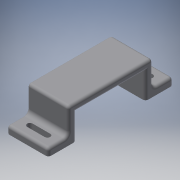
# Autodesk Inventor part: sujeta-taladro-0,1
Saved by Autodesk Inventor 2016 (Build 200138000, 138)
## iProperties
Created: 2015-03-20
Part Number: sujeta-taladro-0,1
Material: Generic
Document SubType Name: Modeling
Designer: pc
Density: 1 g/cm^3
Appearance: Default
Author: pc
Autodesk Inventor part; units mm, degrees
ref_plane "YZ Plane" through (0, 0, 0) normal (1, 0, 0) x (0, 1, 0)
ref_plane "XZ Plane" through (0, 0, 0) normal (0, 1, 0) x (-1, 0, 0)
ref_plane "XY Plane" through (0, 0, 0) normal (0, 0, 1) x (1, 0, 0)
sketch "Sketch1" plane through (0, 0, 0) normal (1, 0, 0) x (0, 1, 0)
  line L0 (-67.5, 3.7308) -> (-37.5, 3.7308)
  line L1 (-37.5, 3.7308) -> (-37.5, 31.7308)
  line L2 (-37.5, 31.7308) -> (37.5, 31.7308)
  line L3 (37.5, 31.7308) -> (37.5, 3.7308)
  line L4 (37.5, 3.7308) -> (67.5, 3.7308)
  line L5 (67.5, 3.7308) -> (67.5, 11.7308)
  line L6 (67.5, 11.7308) -> (45.5, 11.7308)
  line L7 (45.5, 11.7308) -> (45.5, 39.7308)
  line L8 (45.5, 39.7308) -> (-45.5, 39.7308)
  line L9 (-45.5, 39.7308) -> (-45.5, 11.7308)
  line L10 (-45.5, 11.7308) -> (-67.5, 11.7308)
  line L11 (-67.5, 11.7308) -> (-67.5, 3.7308)
  line L12 (0, 0) -> (0, 98)
  dimension "d0" = 75
  dimension "d1" = 30
  dimension "d2" = 8
  dimension "d3" = 8
  dimension "d4" = 8
  dimension "d5" = 8
  dimension "d6" = 28
  constraints: 26 end point, 9 perpendicular, 4 point on line, 1 collinear, 1 horizontal, 1 symmetric about line, 1 vertical
  measures "d0" distance of L1.end L2.end
  measures "d1" distance of L0.start L0.end
  measures "d2" distance from line of L7 L2.end
  measures "d3" distance between parallel lines of L9 L1
  measures "d4" distance between parallel lines of L0 L10
  measures "d5" distance between parallel lines of L2 L8
  measures "d6" distance of L0.end L1.end
extrude "Extrusion1" add sketch "Sketch1" along normal blind 45
sketch "Sketch2" plane through (0, 45.5, 11.7308) normal (0, 0, 1) x (1, 0, 0)
  line L0 (0, -45.5) -> (80, -45.5)
  line L1 (0, 22) -> (0, 0) projected
  line L2 (0, 0) -> (45, 0) projected
  line L3 (45, 22) -> (45, 0) projected
  line L4 (0, 22) -> (45, 22) projected
  line L5 (32, 10) -> (13, 10) construction
  line L6 (32, 7) -> (13, 7)
  line L7 (13, 13) -> (32, 13)
  arc A0 (32, 7) -> (32, 13) centre (32, 10) ccw
  arc A1 (13, 13) -> (13, 7) centre (13, 10) ccw
  line L8 (32, -98) -> (13, -98)
  line L9 (13, -104) -> (32, -104)
  arc A2 (32, -104) -> (32, -98) centre (32, -101) ccw
  arc A3 (13, -98) -> (13, -104) centre (13, -101) ccw
  point P0 (22.5, 10)
  constraints: 14 end point, 8 point on circle, 6 symmetric about line, 4 centre point, 4 tangent, 2 horizontal, 1 midpoint, 1 parallel, 2 other
extrude "Extrusion2" cut sketch "Sketch2" against normal through all contours L6 A1 L7 A0 | A2 L9 A3 L8
fillet "Fillet1" radius 5 2 edges at (22.5, 45.5, 11.7308) (22.5, -45.5, 11.7308)
fillet "Fillet2" radius 3 24 edges at (22.5, 45.5, 39.7308) (0, 0, 39.7308) (0, 37.5, 17.7308) (0, 0, 31.7308) (0, -37.5, 17.7308) (0, -59, 11.7308) (0, -45.5, 28.2308) (45, 0, 39.7308) (45, 59, 11.7308) (45, 45.5, 28.2308) (0, 59, 11.7308) (0, 45.5, 28.2308) (22.5, 67.5, 11.7308) (45, 67.5, 7.7308) (0, 67.5, 7.7308) (22.5, -45.5, 39.7308) (22.5, -67.5, 11.7308) (0, -67.5, 7.7308) (45, -67.5, 7.7308) (45, -59, 11.7308) (45, -45.5, 28.2308) (45, -37.5, 17.7308) (45, 0, 31.7308) (45, 37.5, 17.7308)
body "Solid1"
